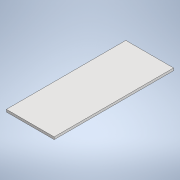
# Autodesk Inventor part: Fan Distribution Case
Saved by Autodesk Inventor 2020 (Build 240168000, 168)
## iProperties
Created: 2019-12-30
Part Number: Fan Distribution Case
Material: Generic
Document SubType Name: Modeling
Designer: pepd9
Density: 1 g/cm^3
Appearance: Default
Author: pepd9
Autodesk Inventor part; units mm, degrees
ref_plane "YZ Plane" through (0, 0, 0) normal (1, 0, 0) x (0, 1, 0)
ref_plane "XZ Plane" through (0, 0, 0) normal (0, 1, 0) x (-1, 0, 0)
ref_plane "XY Plane" through (0, 0, 0) normal (0, 0, 1) x (1, 0, 0)
sketch "Sketch1" plane through (0, 0, 0) normal (0, 1, 0) x (-1, 0, 0)
  line L0 (20, -50) -> (-20, -50)
  line L1 (-20, -50) -> (-20, 50)
  line L2 (-20, 50) -> (20, 50)
  line L3 (20, 50) -> (20, -50)
  line L4 (20, -50) -> (-20, 50) construction
  line L5 (-20, -50) -> (20, 50) construction
  point P0 (0, 0)
  dimension "d0" = 100
  dimension "d1" = 40
  constraints: 12 end point, 2 midpoint, 2 parallel, 1 horizontal, 1 perpendicular
  measures "d0" distance of L0.end L1.end
  measures "d1" distance of L1.end L2.end
extrude "Extrusion1" add sketch "Sketch1" along normal blind 2
sketch "Sketch2" plane through (0, 2, 0) normal (0, 1, 0) x (1, 0, 0)
  line L0 (-10, 42) -> (10, 42)
  line L1 (10, 42) -> (10, 38)
  line L2 (10, 38) -> (-10, 38)
  line L3 (-10, 38) -> (-10, 42)
  line L4 (-10, 42) -> (10, 38) construction
  line L5 (10, 42) -> (-10, 38) construction
  line L6 (-10, -38) -> (10, -38)
  line L7 (10, -38) -> (10, -42)
  line L8 (10, -42) -> (-10, -42)
  line L9 (-10, -42) -> (-10, -38)
  line L10 (-10, -38) -> (10, -42) construction
  line L11 (10, -38) -> (-10, -42) construction
  line L12 (20, -50) -> (20, 50) projected
  line L13 (20, 50) -> (-20, 50) projected
  line L14 (-20, 50) -> (-20, -50) projected
  line L15 (-20, -50) -> (20, -50) projected
  line L16 (-20, 0) -> (20, 0)
  line L17 (20, -50) -> (20, 50) projected
  point P0 (0, 40)
  point P1 (0, -40)
  point P2 (0, 40)
  point P3 (0, 0)
  point P4 (0, 0)
  dimension "d7" = 20
  dimension "d8" = 4
  dimension "d9" = 20
  dimension "d10" = 4
  dimension "d11" = 38
  dimension "d12" = 38
  constraints: 26 end point, 8 midpoint, 4 parallel, 2 horizontal, 2 perpendicular, 2 vertical alignment, 1 coincident
  measures "d7" distance of L1.end L2.end
  measures "d8" distance of L0.end L1.end
  measures "d9" distance of L7.end L8.end
  measures "d10" distance of L6.end L7.end
  measures "d11" distance from line of L2 point (0, 0)
  measures "d12" distance from line of L6 point (0, 0)
extrude "Extrusion2" add sketch "Sketch2" along normal blind 5 contours L0 L1 L2 L3 | L6 L7 L8 L9
sketch "Sketch3" plane through (-10, 2, -42) normal (-1, 0, 0) x (0, 0, 1)
  line L0 (0, 0) -> (0, 5) projected
  line L1 (0, 5) -> (0, 7)
  line L2 (0, 7) -> (2.1, 7)
  line L3 (2.1, 7) -> (1.8, 6.25)
  line L4 (0, 5) -> (4, 5) projected
  line L5 (1.5, 5) -> (0, 5)
  line L6 (1.5, 5) -> (1.8, 5)
  line L7 (1.8, 5) -> (1.8, 6.25)
  point P0 (42, -2)
  dimension "d15" = 2
  dimension "d16" = 2.1
  dimension "d18" = 1.8
  dimension "d19" = 1.25
  constraints: 12 end point, 2 perpendicular, 1 parallel, 1 point on line, 1 vertical
  measures "d15" distance of L0.end L1.end
  measures "d16" distance of L1.end L2.end
  measures "d18" distance between parallel lines of L1 L7
  measures "d19" distance of L6.end L3.end
extrude "Extrusion3" add sketch "Sketch3" against normal up to surface (20 mm away)
mirror "Mirror1" about plane through (0, 0, 0) normal (0, 0, 1) of "Extrusion3"
sketch "Sketch4" plane through (0, 2, 0) normal (0, 1, 0) x (1, 0, 0)
  line L0 (12.3, 15) -> (10.3, 15)
  line L1 (10.3, 15) -> (10.3, -15)
  line L2 (10.3, -15) -> (12.3, -15)
  line L3 (12.3, -15) -> (12.3, 15)
  line L4 (12.3, 15) -> (10.3, -15) construction
  line L5 (10.3, 15) -> (12.3, -15) construction
  line L6 (-10.3, 15) -> (-12.3, 15)
  line L7 (-12.3, 15) -> (-12.3, -15)
  line L8 (-12.3, -15) -> (-10.3, -15)
  line L9 (-10.3, -15) -> (-10.3, 15)
  line L10 (-10.3, 15) -> (-12.3, -15) construction
  line L11 (-12.3, 15) -> (-10.3, -15) construction
  point P0 (0, 0)
  point P1 (11.3, 0)
  point P2 (-11.3, 0)
  point P3 (11.3, 0)
  point P4 (-11.3, 0)
  dimension "d22" = 30
  dimension "d23" = 30
  dimension "d24" = 2
  dimension "d25" = 2
  dimension "d26" = 10.3
  dimension "d27" = 10.3
  constraints: 24 end point, 6 midpoint, 4 parallel, 2 horizontal, 2 horizontal alignment, 2 perpendicular
  measures "d22" distance of L2.end L0.start
  measures "d23" distance of L6.end L7.end
  measures "d24" distance of L6.start L6.end
  measures "d25" distance of L0.start L0.end
  measures "d26" distance from line of L1 point (0, 0)
  measures "d27" distance from line of L9 point (0, 0)
extrude "Extrusion4" add sketch "Sketch4" along normal blind 7
chamfer "Chamfer1" distance 5 angle 45 4 edges at (-11.3, 2, 15) (-11.3, 2, -15) (11.3, 2, -15) (11.3, 2, 15)
chamfer "Chamfer2" distance 5 angle 20 3 edges at (-12.3, 2, 17.5) (-12.3, 2, 0) (-12.3, 2, -17.5) measured on face at (-12.3, 2.5, 0) measured on face at (-12.3, 2.5, 17.5) measured on face at (-12.3, 2.5, -17.5)
chamfer "Chamfer3" distance 5 angle 20 3 edges at (12.3, 2, -17.5) (12.3, 2, 0) (12.3, 2, 17.5) measured on face at (12.3, 2.5, -17.5) measured on face at (12.3, 2.5, 0) measured on face at (12.3, 2.5, 17.5)
sketch "Sketch5" plane through (0, 2, 0) normal (0, 1, 0) x (1, 0, 0)
  circle A0 centre (-24, 50) radius 4
  circle A1 centre (-24, -50) radius 4
  line L0 (-20, 50) -> (-20, -50) projected
  line L1 (-20, -50) -> (20, -50) projected
  line L2 (-24.6587, 53.9454) -> (0, 50)
  line L3 (20, 50) -> (-20, 50) projected
  line L4 (-28, -50) -> (-20, 0)
  line L5 (-28, 50) -> (-20, 0)
  line L6 (-24, -54) -> (0, -50)
  point P0 (0, 0)
  dimension "d39" = 8
  dimension "d40" = 8
  dimension "d41" = 100
  dimension "d42" = 4
  dimension "d43" = 0
  constraints: 8 end point, 4 point on circle, 3 midpoint, 2 centre point, 1 perpendicular, 1 vertical alignment
  measures "d39" diameter of A0
  measures "d40" diameter of A1
  measures "d41" distance of A1.centre A0.centre
  measures "d42" distance from line of L0 A1.centre
  measures "d43" distance from line of L1 A1.centre
extrude "Extrusion5" add sketch "Sketch5" against normal up to surface (2 mm away) contours L2 A0 L5 | L0 A1 L4 | L2 L3 A0 | A0 L0 L5 | A1 L6 L4 | L1 L6 A1
sketch "Sketch6" plane through (0, 2, 0) normal (0, 1, 0) x (1, 0, 0)
  arc A0 (-24.6587, 53.9454) -> (-28, 50) centre (-24, 50) ccw projected
  arc A1 (-28, -50) -> (-24, -54) centre (-24, -50) ccw projected
  point P0 (0, 0)
hole "Hole1" at (-24, 2, -50) at (-24, 2, 50) direction (0, -1, 0) diameter 3.4 end through all clearance for "Socket Head Cap Screw" size "M3" standard "Ansi Metric M Profile"
chamfer "Chamfer4" distance 15 angle 45 1 edges at (20, 1, 50)
sketch "Sketch7" plane through (0, 2, 0) normal (0, 1, 0) x (1, 0, 0)
  line L0 (20, -35) -> (5, -50) projected
  line L1 (20, -35) -> (20, 50) projected
  line L2 (20, 50) -> (0, 50) projected
  line L3 (0, 50) -> (-24.6587, 53.9454) projected
  arc A0 (-24.6587, 53.9454) -> (-28, 50) centre (-24, 50) ccw projected
  line L4 (-28, 50) -> (-20, 0) projected
  line L5 (-20, 0) -> (-28, -50) projected
  arc A1 (-28, -50) -> (-24, -54) centre (-24, -50) ccw projected
  line L6 (-24, -54) -> (0, -50) projected
  line L7 (0, -50) -> (5, -50) projected
  line L8 (-10, 38) -> (-10, 42) projected
  line L9 (-10, 42) -> (10, 42) projected
  line L10 (10, 42) -> (10, 38) projected
  line L11 (10, 38) -> (-10, 38) projected
  line L12 (10, -38) -> (10, -42) projected
  line L13 (10, -42) -> (-10, -42) projected
  line L14 (-10, -42) -> (-10, -38) projected
  line L15 (-10, -38) -> (10, -38) projected
  line L16 (-10.3, 20) -> (-14.1199, 20) projected
  line L17 (-10.3, 20) -> (-10.3, -20) projected
  line L18 (-14.1199, -20) -> (-10.3, -20) projected
  line L19 (-14.1199, 20) -> (-14.1199, -20) projected
  line L20 (10.3, -20) -> (14.1199, -20) projected
  line L21 (10.3, -20) -> (10.3, 20) projected
  line L22 (14.1199, 20) -> (10.3, 20) projected
  line L23 (14.1199, -20) -> (14.1199, 20) projected
  circle A2 centre (-24, -50) radius 1.7 projected
  circle A3 centre (-24, 50) radius 1.7 projected
  line L24 (18, 50) -> (18, -34.1716)
  line L25 (18, -34.1716) -> (4.1716, -48)
  line L26 (4.1716, -48) -> (-0.1655, -48)
  line L27 (-24.6587, 53.9454) -> (0, 50) projected
  line L28 (0, 50) -> (-18.3194, 50)
  line L29 (-18.3194, 50) -> (-18.3194, -50)
  line L30 (-18.3194, -50) -> (0, -50)
  line L31 (-0.1655, -48) -> (-16.3194, -48)
  line L32 (-16.3194, -48) -> (-16.3194, 50)
  point P0 (0, 0)
  dimension "d56" = 2
  dimension "d57" = 2
  dimension "d58" = 2
  constraints: 16 end point, 3 perpendicular, 2 horizontal, 2 point on line, 1 other
  measures "d56" distance between parallel lines of L1 L24
  measures "d57" distance between parallel lines of L30 L31
  measures "d58" distance between parallel lines of L29 L32
extrude "Extrusion6" add sketch "Sketch7" along normal blind 20 contours L0 L7 L30 L29 L28 L32 L31 L26 L25 L24 L2 L1
ref_plane "Work Plane1" through (0, 0, 0) normal (0, 0, 1) x (1, 0, 0)
body "Solid1"
